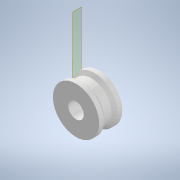
# Autodesk Inventor part: kółko
Saved by Autodesk Inventor 2022.3 (Build 263350000, 350)
## iProperties
Created: 2022-12-14
Part Number: kółko
Material: Generic
Document SubType Name: Modeling
Designer: komputer
Density: 1 g/cm^3
Appearance: Default
Author: komputer
Autodesk Inventor part; units mm, degrees
ref_plane "YZ Plane" through (0, 0, 0) normal (1, 0, 0) x (0, 1, 0)
ref_plane "XZ Plane" through (0, 0, 0) normal (0, 1, 0) x (-1, 0, 0)
ref_plane "XY Plane" through (0, 0, 0) normal (0, 0, 1) x (1, 0, 0)
sketch "Sketch1" plane through (0, 0, 0) normal (0, 0, 1) x (1, 0, 0)
  circle A0 centre (0, 0) radius 1 projected
  circle A1 centre (0, 0) radius 1 projected
  circle A2 centre (0, 0) radius 3 projected
  line L0 (0, -1) -> (0, -3)
  circle A3 centre (0, 0) radius 3
  dimension "d0" = 2
  constraints: 3 vertical alignment, 2 end point, 1 coincident, 4 other
  measures "d0" distance of L0.start L0.end
extrude "Extrusion1" add sketch "Sketch1" against normal blind 3
ref_plane "Work Plane1" through (-3.9635, 7.3942, -4.6) normal (-0.9999878, 0.0049495, 0) x (0.0049495, 0.9999878, 0)
sketch "Sketch2" plane through (-3.9635, 7.3942, -4.6) normal (-0.9999878, 0.0049495, 0) x (0.0049495, 0.9999878, 0)
  line L0 (-4.3745, -1.6) -> (-10.3745, -1.6) projected
  line L1 (-10.3745, -4.6) -> (-4.3745, -4.6) projected
  line L2 (-8.3745, -1.6) -> (-8.3745, -4.6) projected
  line L3 (-5.7, -1) -> (-5.7, -4.6)
  line L4 (-10.3745, -4.6) -> (-4.3745, -4.6) projected
  line L5 (-10.3745, -4.6) -> (-10.3745, -1.6)
  line L6 (-10.3745, -4.6) -> (-10.3745, -1.6) projected
  line L7 (-10.3745, -3.1) -> (-9.2989, -3.1)
  line L8 (-9.2989, -3.1) -> (-9.2989, -2.6)
  line L9 (-9.2989, -2.6) -> (-9.2989, -3.6)
  line L10 (-9.2989, -3.6) -> (-10.3745, -3.6)
  line L11 (-9.2989, -3.6) -> (-10.3745, -4.0041)
  line L12 (-9.2989, -3.6) -> (-9.2989, -2.6)
  line L13 (-9.2989, -2.6) -> (-10.3745, -2.1959)
  point P0 (-7.3745, -4.6)
  point P1 (-10.3745, -2.1959)
  dimension "d3" = 0.5
  dimension "d4" = 1
  constraints: 18 end point, 3 point on line, 3 symmetric about line, 2 vertical, 1 collinear, 1 horizontal, 1 midpoint, 1 perpendicular, 2 other
  measures "d3" distance of L7.end L8.end
  measures "d4" distance of L8.end L9.end
extrude "Extrusion2" cut sketch "Sketch2" against normal through all contours L13 L8 L7 L5 | L7 L9 L10 L5 | L5 L10 L11
pattern_circular "Circular Pattern1" count 40 over 360 about axis through (0, 0, 0) along (0, 0, -1) of "Extrusion2"
body "Solid1"
